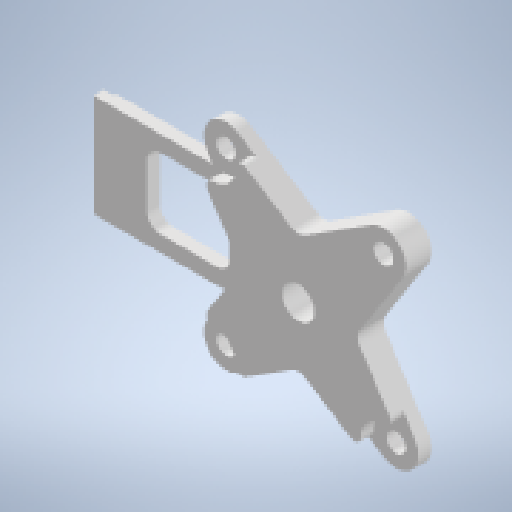
# Autodesk Inventor part: TurretBase
Saved by Autodesk Inventor 2023 (Build 270158000, 158)
## iProperties
Created: 2023-05-07
Part Number: TurretBase
Material: Generic
Document SubType Name: Modeling
Designer: karpova
Density: 1 g/cm^3
Appearance: Default
Author: karpova
Autodesk Inventor part; units mm, degrees
ref_plane "YZ Plane" through (0, 0, 0) normal (1, 0, 0) x (0, 1, 0)
ref_plane "XZ Plane" through (0, 0, 0) normal (0, 1, 0) x (-1, 0, 0)
sketch "Sketch1" plane through (0, 0, 0) normal (0, 0, 1) x (1, 0, 0)
  line L0 (-1.5875, 0) -> (-1.5875, -108.1) projected
  line L1 (-54.875, 0) -> (-1.5875, 0) projected
  line L2 (-54.875, 0) -> (-54.875, -59) projected
  line L3 (-54.875, -59) -> (-18.9375, -59) projected
  arc A0 (-18.9375, -75) -> (-18.9375, -59) centre (-18.9375, -67) ccw projected
  line L4 (-18.9375, -75) -> (-54.875, -75) projected
  line L5 (-54.875, -75) -> (-54.875, -108.1) projected
  line L6 (-54.875, -108.1) -> (-1.5875, -108.1) projected
  circle A1 centre (-18.9375, -67) radius 2 projected
  circle A2 centre (-18.9375, -67) radius 2 projected
  circle A3 centre (-18.9375, -67) radius 7.5 projected
  line L7 (-6.1875, -79.75) -> (-31.6875, -79.75) construction
  line L8 (-31.6875, -79.75) -> (-31.6875, -54.25) construction
  line L9 (-31.6875, -54.25) -> (-6.1875, -54.25) construction
  line L10 (-6.1875, -54.25) -> (-6.1875, -79.75) construction
  line L11 (-18.9375, -79.75) -> (-18.9375, -54.25) construction
  line L12 (-31.6875, -67) -> (-6.1875, -67) construction
  circle A4 centre (-6.1875, -79.75) radius 1.5
  circle A5 centre (-31.6875, -79.75) radius 1.5
  circle A6 centre (-31.6875, -54.25) radius 1.5
  circle A7 centre (-6.1875, -54.25) radius 1.5
  circle A8 centre (-6.1875, -79.75) radius 2.6 construction
  circle A9 centre (-31.6875, -79.75) radius 2.6 construction
  circle A10 centre (-31.6875, -54.25) radius 2.6 construction
  circle A11 centre (-6.1875, -54.25) radius 2.6 construction
  line L13 (-3.5875, -79.75) -> (-3.5875, -54.25) construction
  arc A12 (-8.0517, -82.7122) -> (-3.5875, -77.4069) centre (-6.1875, -79.75) ccw
  arc A13 (-34.6497, -77.8858) -> (-29.8233, -82.7122) centre (-31.6875, -79.75) ccw
  arc A14 (-29.8233, -51.2878) -> (-34.6497, -56.1142) centre (-31.6875, -54.25) ccw
  arc A15 (-3.5875, -56.5931) -> (-8.0517, -51.2878) centre (-6.1875, -54.25) ccw
  line L14 (-8.0517, -82.7122) -> (-17.8722, -76.532)
  line L15 (-34.6497, -56.1142) -> (-28.4695, -65.9347)
  line L16 (-34.6497, -77.8858) -> (-28.4695, -68.0653)
  line L17 (-3.2253, -56.1142) -> (-9.4055, -65.9347)
  line L18 (-3.2253, -77.8858) -> (-9.4055, -68.0653)
  line L19 (-29.8233, -51.2878) -> (-20.0028, -57.468)
  line L20 (-8.0517, -51.2878) -> (-17.8722, -57.468)
  line L21 (-20.3773, -59) -> (-20.6867, -59.1936)
  line L22 (-29.8233, -82.7122) -> (-20.0028, -76.532)
  arc A16 (-20.0028, -57.468) -> (-17.8722, -57.468) centre (-18.9375, -55.7753) ccw
  arc A17 (-28.4695, -68.0653) -> (-28.4695, -65.9347) centre (-30.1622, -67) ccw
  arc A18 (-17.8722, -76.532) -> (-20.0028, -76.532) centre (-18.9375, -78.2247) ccw
  arc A19 (-9.4055, -65.9347) -> (-9.4055, -68.0653) centre (-7.7128, -67) ccw
  circle A20 centre (-18.9375, -67) radius 2.5
  circle A21 centre (-31.6875, -54.25) radius 2.6 projected
  circle A22 centre (-6.1875, -79.75) radius 2.6 projected
  circle A23 centre (-6.1875, -54.25) radius 2.6 projected
  circle A24 centre (-31.6875, -79.75) radius 2.6 projected
  point P0 (0, 0)
  point P1 (-27.7991, -67)
  point P2 (-10.0759, -67)
  point P3 (-18.9375, -58.1384)
  point P4 (-18.9375, -75.8616)
  dimension "d2" = 5.2
  dimension "d1" = 3
  dimension "d4" = 2
  dimension "d5" = 2
  dimension "d6" = 2
  dimension "d9" = 0.5
  constraints: 32 end point, 19 point on circle, 18 tangent, 15 centre point, 15 point on line, 14 coincident, 10 equal radius, 5 midpoint, 5 perpendicular, 4 horizontal alignment, 3 parallel, 1 horizontal, 1 vertical, 6 other
  measures "d1" diameter of A4
  measures "d4" distance between parallel lines of L0 L13
  measures "d5" radial gap between concentric circles of A12 A4
  measures "d6" radius of A16
  measures "d9" radial gap between concentric circles of A20 A1
extrude "Extrusion1" add sketch "Sketch1" along normal blind 4 contours L15 A14 L19 A16 L20 A15 L17 A19 L18 A12 L14 A18 L22 A13 L16 L4 A0 L3 | L3 A0 L4 L16 A17 L15 | A3 | A21 | A22 | A23 | A24
sketch "Sketch2" plane through (0, 0, 0) normal (0, 0, -1) x (-1, 0, 0)
  circle A0 centre (18.9375, -67) radius 7.5 projected
  point P0 (0, 0)
extrude "Extrusion2" add sketch "Sketch2" along normal blind 1
sketch "Sketch3" plane through (0, 0, 0) normal (0, 0, -1) x (-1, 0, 0)
  line L0 (1.5875, 0) -> (1.5875, -108.1) projected
  line L1 (54.875, 0) -> (1.5875, 0) projected
  line L2 (54.875, 0) -> (54.875, -59) projected
  line L3 (54.875, -59) -> (18.9375, -59) projected
  arc A0 (18.9375, -59) -> (18.9375, -75) centre (18.9375, -67) ccw projected
  line L4 (18.9375, -75) -> (54.875, -75) projected
  line L5 (54.875, -75) -> (54.875, -108.1) projected
  line L6 (54.875, -108.1) -> (1.5875, -108.1) projected
  circle A1 centre (18.9375, -67) radius 7.5 projected
  arc A2 (18.9375, -59) -> (18.9375, -75) centre (18.9375, -67) ccw projected
  circle A3 centre (18.9375, -67) radius 2.5 projected
  arc A4 (22.7022, -74.0588) -> (22.7022, -59.9412) centre (18.9375, -67) ccw
  line L7 (53.2875, -108.1) -> (53.2875, 0) projected
  line L8 (54.875, 0) -> (54.875, -108.1) projected
  line L9 (53.2875, -59) -> (22.9375, -59)
  line L10 (18.9375, -59) -> (18.9375, -75)
  line L11 (22.9375, -75) -> (53.2875, -75)
  line L12 (53.2875, -75) -> (53.2875, -59)
  arc A5 (22.9375, -59) -> (22.7022, -59.9412) centre (22.9375, -59.5) ccw
  arc A6 (22.7022, -74.0588) -> (22.9375, -75) centre (22.9375, -74.5) ccw
  circle A7 centre (31.6875, -54.25) radius 2.6 projected
  circle A8 centre (6.1875, -79.75) radius 2.6 projected
  circle A9 centre (6.1875, -54.25) radius 2.6 projected
  circle A10 centre (31.6875, -79.75) radius 2.6 projected
  point P0 (0, 0)
  dimension "d12" = 0.5
  constraints: 9 point on circle, 8 end point, 4 point on line, 4 tangent, 3 centre point, 2 parallel, 1 coincident, 1 equal radius, 1 horizontal, 1 perpendicular
  measures "d12" radius of A5
extrude "Extrusion3" add sketch "Sketch3" along normal blind 2 contours L7 L4 A6 A4 A5 L3
sketch "Sketch4" plane through (-53.2875, -75, 0) normal (-1, 0, 0) x (0, 0, 1)
  line L0 (-1.5875, 75) -> (-1.5875, -33.1) projected
  line L1 (0, -33.1) -> (0, 75) projected
  line L2 (0, 15.0588) -> (0, 16) projected
  line L3 (0, 0) -> (-2, 0) projected
  line L4 (0, 16) -> (-1.5875, 16)
  line L5 (-1.5875, 16) -> (-1.5875, 0)
  line L6 (-1.5875, 0) -> (0, 0)
  line L7 (0, 0) -> (0, 16)
  constraints: 8 end point, 2 parallel, 2 point on line, 1 horizontal, 1 perpendicular
ref_plane "Work Plane1" through (-54.875, -108.1, -1.5875) normal (1, 0, 0) x (0, 1, 0)
extrude "Extrusion4" add sketch "Sketch4" along normal up to surface (1.5875 mm away)
sketch "Sketch5" plane through (0, 0, 4) normal (0, 0, 1) x (1, 0, 0)
  arc A0 (-28.4695, -68.0653) -> (-28.4695, -65.9347) centre (-30.1622, -67) ccw projected
  line L0 (-28.4695, -68.0653) -> (-34.6497, -77.8858) projected
  arc A1 (-34.6497, -77.8858) -> (-29.8233, -82.7122) centre (-31.6875, -79.75) ccw projected
  line L1 (-29.8233, -82.7122) -> (-20.0028, -76.532) projected
  arc A2 (-17.8722, -76.532) -> (-20.0028, -76.532) centre (-18.9375, -78.2247) ccw projected
  line L2 (-17.8722, -76.532) -> (-8.0517, -82.7122) projected
  arc A3 (-8.0517, -82.7122) -> (-3.2253, -77.8858) centre (-6.1875, -79.75) ccw projected
  line L3 (-3.2253, -77.8858) -> (-9.4055, -68.0653) projected
  arc A4 (-9.4055, -65.9347) -> (-9.4055, -68.0653) centre (-7.7128, -67) ccw projected
  line L4 (-9.4055, -65.9347) -> (-3.2253, -56.1142) projected
  arc A5 (-3.2253, -56.1142) -> (-8.0517, -51.2878) centre (-6.1875, -54.25) ccw projected
  line L5 (-8.0517, -51.2878) -> (-17.8722, -57.468) projected
  arc A6 (-20.0028, -57.468) -> (-17.8722, -57.468) centre (-18.9375, -55.7753) ccw projected
  line L6 (-20.0028, -57.468) -> (-29.8233, -51.2878) projected
  arc A7 (-29.8233, -51.2878) -> (-34.6497, -56.1142) centre (-31.6875, -54.25) ccw projected
  line L7 (-34.6497, -56.1142) -> (-28.4695, -65.9347) projected
  circle A8 centre (-18.9375, -67) radius 2.5 projected
  circle A9 centre (-6.1875, -54.25) radius 1.5 projected
  circle A10 centre (-31.6875, -54.25) radius 1.5 projected
  circle A11 centre (-31.6875, -79.75) radius 1.5 projected
  circle A12 centre (-6.1875, -79.75) radius 1.5 projected
  circle A13 centre (-31.6875, -79.75) radius 3.5
  circle A14 centre (-31.6875, -54.25) radius 1.5 projected
  circle A15 centre (-31.6875, -54.25) radius 3.5
  circle A16 centre (-6.1875, -79.75) radius 3.5
  arc A17 (-3.2253, -56.1142) -> (-8.0517, -51.2878) centre (-6.1875, -54.25) ccw projected
  circle A18 centre (-6.1388, -54.2188) radius 3.5
  point P0 (0, 0)
  point P1 (-34.6497, -56.1142)
  point P2 (-29.8233, -51.2878)
  point P3 (-2.2565, -55.1629)
  point P4 (-3.2253, -77.8858)
  point P5 (-8.0517, -82.7122)
  point P6 (-29.8233, -82.7122)
  point P7 (-3.4179, -56.4203)
  constraints: 3 centre point, 3 coincident, 3 concentric, 3 other
extrude "Extrusion5" cut sketch "Sketch5" against normal blind 2 contours A13 A1 | A7 A15 | A16 A3 | A5 L4 A18 picked at (-4.1737, -56.2279)
fillet "Fillet1" radius 1 10 edges at (-8.0517, -82.7122, 3) (-3.2253, -77.8858, 3) (-3.2253, -56.1142, 1) (-8.0517, -51.2878, 1) (-29.8233, -51.2878, 3) (-34.6497, -56.1142, 3) (-34.6497, -77.8858, 3) (-29.8233, -82.7122, 3) (-3.4179, -56.4203, 3) (-8.0517, -51.2878, 3)
sketch "Sketch6" plane through (0, 0, 0) normal (0, 0, 1) x (1, 0, 0)
  line L0 (-32.8336, -59) -> (-28.4695, -65.9347) projected
  line L1 (-32.8336, -59) -> (-54.875, -59) projected
  line L2 (-54.875, -75) -> (-54.875, -59) projected
  line L3 (-32.8336, -75) -> (-54.875, -75) projected
  line L4 (-28.4695, -68.0653) -> (-32.8336, -75) projected
  arc A0 (-28.4695, -68.0653) -> (-28.4695, -65.9347) centre (-30.1622, -67) ccw projected
  line L5 (-53.2875, 0) -> (-53.2875, -108.1) projected
  line L6 (-35.6304, -72.5101) -> (-44.525, -72.5101)
  line L7 (-46.525, -70.5101) -> (-46.525, -63.4899)
  line L8 (-44.525, -61.4899) -> (-35.6304, -61.4899)
  line L9 (-33.6304, -63.4899) -> (-33.6304, -70.5101)
  line L10 (-28.1622, -67) -> (-54.875, -67) construction
  line L11 (-54.875, -59) -> (-54.875, -75) construction
  line L12 (-48.525, -39.75) -> (-48.525, -93.75) construction
  arc A1 (-35.6304, -72.5101) -> (-33.6304, -70.5101) centre (-35.6304, -70.5101) ccw
  arc A2 (-46.525, -70.5101) -> (-44.525, -72.5101) centre (-44.525, -70.5101) ccw
  arc A3 (-44.525, -61.4899) -> (-46.525, -63.4899) centre (-44.525, -63.4899) ccw
  arc A4 (-33.6304, -63.4899) -> (-35.6304, -61.4899) centre (-35.6304, -63.4899) ccw
  point P0 (0, 0)
  dimension "d20" = 2
  dimension "d21" = 2
  constraints: 10 end point, 9 point on circle, 8 tangent, 4 centre point, 3 equal radius, 2 parallel, 1 horizontal, 1 midpoint, 1 perpendicular, 1 other
  measures "d20" distance between parallel lines of L12 L7
  measures "d21" radius of A1
extrude "Extrusion6" cut sketch "Sketch6" against normal through all contours L6 A2 L7 A3 L8 A4 L9 A1
body "Solid1"
